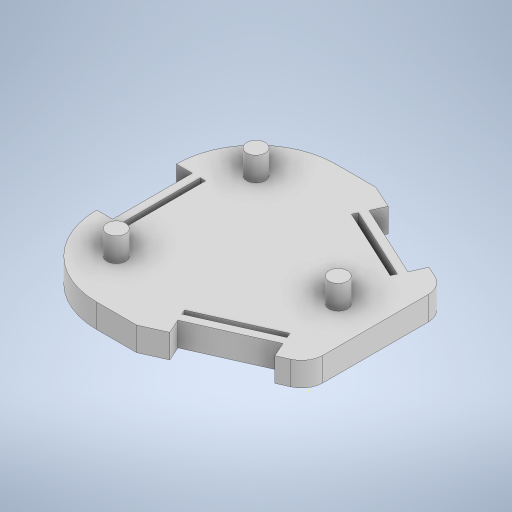
# Autodesk Inventor part: palm
Saved by Autodesk Inventor 2024.3 (Build 283343000, 343)
## iProperties
Created: 2024-11-16
Part Number: palm
Material: Generic
Document SubType Name: Modeling
Designer: Ryba
Density: 1 g/cm^3
Appearance: Default
Author: Ryba
Autodesk Inventor part; units mm, degrees
ref_plane "YZ Plane" through (0, 0, 0) normal (1, 0, 0) x (0, 1, 0)
ref_plane "XZ Plane" through (0, 0, 0) normal (0, 1, 0) x (-1, 0, 0)
ref_plane "XY Plane" through (0, 0, 0) normal (0, 0, 1) x (1, 0, 0)
sketch "Sketch1" plane through (0, 0, 0) normal (0, 1, 0) x (-1, 0, 0)
  line L0 (0, 0) -> (0, -50)
  line L1 (90, -50) -> (90, 0)
  line L2 (90, -25) -> (90, -70)
  line L3 (90, -25) -> (90, 20)
  line L4 (90, 20) -> (60, 20)
  line L5 (90, -70) -> (60, -70)
  line L6 (60, 20) -> (45, 20)
  line L7 (60, -70) -> (45, -70)
  line L8 (45, -70) -> (0, -50)
  line L9 (45, 20) -> (0, 0)
  constraints: 20 end point, 4 horizontal, 2 vertical, 1 midpoint, 1 point on line
extrude "Extrusion1" add sketch "Sketch1" along normal blind 9
fillet "Fillet1" radius 30 2 edges at (-90, 4.5, 20) (-90, 4.5, -70)
sketch "Sketch2" plane through (0, 9, 0) normal (0, 1, 0) x (1, 0, 0)
  arc A0 (-90, 10) -> (-60, -20) centre (-60, 10) ccw projected
  line L0 (-90, 10) -> (-84, 10)
  line L1 (-90, 40) -> (-90, 10) projected
  line L2 (-90, 40) -> (-84, 40)
  line L3 (-84, 40) -> (-84, 10)
  line L4 (-45, -20) -> (0, 0) projected
  line L5 (-45, -20) -> (-22.6116, -10.0496)
  line L6 (-22.6116, -10.0496) -> (-36.3188, -16.1417)
  line L7 (-22.6116, -10.0496) -> (-8.9044, -3.9575)
  line L8 (-8.9044, -3.9575) -> (-11.3413, 1.5253)
  line L9 (-36.3188, -16.1417) -> (-38.7556, -10.6588)
  line L10 (-38.7556, -10.6588) -> (-11.3413, 1.5253)
  line L11 (0, 50) -> (-45, 70) projected
  line L12 (-45, 70) -> (-22.6116, 60.0496)
  line L13 (-22.6116, 60.0496) -> (-36.3188, 66.1417)
  line L14 (-36.3188, 66.1417) -> (-38.7556, 60.6588)
  line L15 (-22.5, 60) -> (-8.7928, 53.9079)
  line L16 (-8.7928, 53.9079) -> (-11.2297, 48.4251)
  line L17 (-11.2297, 48.4251) -> (-38.5472, 61.1277)
  dimension "d11" = 6
  constraints: 30 end point, 7 point on line, 6 perpendicular, 2 horizontal, 1 midpoint
  measures "d11" distance of L0.start L0.end
extrude "Extrusion2" cut sketch "Sketch2" against normal blind 9
fillet "Fillet2" radius 8 2 edges at (0, 4.5, 0) (0, 4.5, -50)
sketch "Sketch3" plane through (0, 9, 0) normal (0, 1, 0) x (1, 0, 0)
  line L0 (-84, 40) -> (-84, 10) projected
  line L1 (-81, 10) -> (-81, 40)
  line L2 (-81, 40) -> (-79, 40)
  line L3 (-79, 40) -> (-79, 10)
  line L4 (-79, 10) -> (-81, 10)
  line L5 (-36.3188, -16.1417) -> (-38.7556, -10.6588) projected
  line L6 (-39.974, -7.9174) -> (-12.5597, 4.2668)
  line L7 (-12.5597, 4.2668) -> (-13.372, 6.0944)
  line L8 (-13.372, 6.0944) -> (-40.7863, -6.0898)
  line L9 (-40.7863, -6.0898) -> (-39.974, -7.9174)
  line L10 (-38.5472, 61.1277) -> (-38.7617, 60.6665)
  line L11 (-11.2297, 48.4251) -> (-38.5472, 61.1277) projected
  line L12 (-39.8122, 58.4074) -> (-12.4946, 45.7048)
  line L13 (-12.4946, 45.7048) -> (-13.3379, 43.8912)
  line L14 (-13.3379, 43.8912) -> (-40.6555, 56.5938)
  line L15 (-40.6555, 56.5938) -> (-39.8122, 58.4074)
  point P0 (0, 0)
  constraints: 26 end point, 8 perpendicular, 1 point on line
extrude "Extrusion3" cut sketch "Sketch3" against normal blind 9
sketch "Sketch4" plane through (0, 9, 0) normal (0, 1, 0) x (1, 0, 0)
  arc A0 (-90, 10) -> (-60, -20) centre (-60, 10) ccw projected
  line L0 (-60, 10) -> (-81.2132, -11.2132)
  line L1 (-60, 10) -> (-30, 10) construction
  arc A1 (-60, 70) -> (-90, 40) centre (-60, 40) ccw projected
  line L2 (-60, 40) -> (-78.753, 58.753)
  line L3 (-60, 40) -> (-33.4792, 40) construction
  line L4 (0, 5.199) -> (0, 44.801) projected
  line L5 (0, 25) -> (-14, 25)
  line L6 (-81.2132, -11.2132) -> (-71.3137, -1.3137)
  line L7 (-81.2132, 61.2132) -> (-71.3137, 51.3137)
  circle A2 centre (-71.3137, -1.3137) radius 3.5
  circle A3 centre (-71.3137, 51.3137) radius 3.5
  circle A4 centre (-14, 25) radius 3.5
  point P0 (0, 0)
  dimension "d38" = 7
  dimension "d39" = 7
  dimension "d40" = 7
  constraints: 14 end point, 3 centre point, 3 coincident, 3 horizontal, 2 equal length, 2 point on circle, 2 point on line, 1 midpoint
  measures "d38" diameter of A2
  measures "d39" diameter of A3
  measures "d40" diameter of A4
extrude "Extrusion4" add sketch "Sketch4" along normal blind 9
sketch "Sketch5" plane through (0, 0, 0) normal (0, -1, 0) x (1, 0, 0)
  point P0 (0, 0)
body "Solid1"
